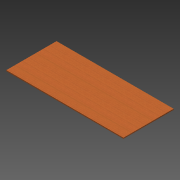
# Autodesk Inventor part: top-plate
Saved by Autodesk Inventor 2013 (Build 170138000, 138)
## iProperties
Created: 2013-05-01
Part Number: top-plate
Material: Wood (Cherry)
Document SubType Name: Modeling
Designer: Chris
Density: 1 g/cm^3
Author: Chris
Autodesk Inventor part; units mm, degrees
ref_plane "YZ Plane" through (0, 0, 0) normal (1, 0, 0) x (0, 1, 0)
ref_plane "XZ Plane" through (0, 0, 0) normal (0, 1, 0) x (-1, 0, 0)
ref_plane "XY Plane" through (0, 0, 0) normal (0, 0, 1) x (1, 0, 0)
sketch "Sketch1" plane through (0, 0, 0) normal (0, 1, 0) x (-1, 0, 0)
  line L0 (0, 0) -> (1422.4, 0)
  line L1 (1422.4, 0) -> (1422.4, 609.6)
  line L2 (1422.4, 609.6) -> (0, 609.6)
  line L3 (0, 609.6) -> (0, 0)
  line L4 (19.05, 596.9) -> (1403.35, 596.9)
  line L5 (1403.35, 596.9) -> (1403.35, 566.0898)
  line L6 (1403.35, 566.0898) -> (19.05, 566.0898)
  line L7 (19.05, 566.0898) -> (19.05, 596.9)
  line L8 (711.2, 596.9) -> (711.2, 566.0898)
  line L9 (711.2, 0) -> (711.2, 609.6)
  dimension "d0" = 1422.4
  dimension "d1" = 609.6
  dimension "d4" = 30.8102
  dimension "d6" = 1384.3
  dimension "d7" = 12.7
  constraints: 20 end point, 4 midpoint, 4 parallel, 2 horizontal, 2 perpendicular, 1 collinear
  measures "d0" distance of L2.end L1.end
  measures "d1" distance of L1.end L0.end
  measures "d4" distance of L4.end L5.end
  measures "d6" distance of L5.end L6.end
  measures "d7" distance between parallel lines of L2 L4
extrude "Extrusion1" add sketch "Sketch1" along normal blind 12.7
body "Solid1"
